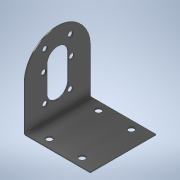
# Autodesk Inventor part: motorBracket
Saved by Autodesk Inventor 2020 (Build 240168000, 168)
## iProperties
Created: 2022-07-22
Part Number: motorBracket
Material: Aluminum 6061
Document SubType Name: Sheet Metal
Designer: iPICLab4
Density: 2.7 g/cm^3
Sheet Metal Rule: Default_mm
Appearance: Dark Gray
Author: iPICLab4
Autodesk Inventor part; units mm, degrees
ref_plane "YZ Plane" through (0, 0, 0) normal (1, 0, 0) x (0, 1, 0)
ref_plane "XZ Plane" through (0, 0, 0) normal (0, 1, 0) x (-1, 0, 0)
ref_plane "XY Plane" through (0, 0, 0) normal (0, 0, 1) x (1, 0, 0)
sketch "Sketch1" plane through (0, 0, 0) normal (0, 1, 0) x (-1, 0, 0)
  line L0 (0, 0) -> (67, 0)
  line L1 (67, -40) -> (0, -40)
  line L2 (0, -40) -> (0, 0)
  line L3 (40, 0) -> (40, -40)
  circle A0 centre (30, -5) radius 1.75
  circle A1 centre (30, -35) radius 1.75
  circle A2 centre (10, -5) radius 1.75
  circle A3 centre (10, -35) radius 1.75
  line L4 (55, -20) -> (70, -20) construction
  line L5 (55, -13.5) -> (70, -13.5)
  line L6 (70, -26.5) -> (55, -26.5)
  arc A4 (55, -13.5) -> (55, -26.5) centre (55, -20) ccw
  arc A5 (70, -26.5) -> (70, -13.5) centre (70, -20) ccw
  circle A6 centre (67, -28.5) radius 1.5
  circle A7 centre (67, -11.5) radius 1.5
  circle A8 centre (50, -27.75) radius 1.5
  circle A9 centre (79, -12.25) radius 1.5
  circle A10 centre (79, -27.75) radius 1.5
  circle A11 centre (50, -12.25) radius 1.5
  arc A12 (67, -40) -> (67, 0) centre (67, -20) ccw
  point P0 (62.5, -20)
  dimension "d1" = 40
  dimension "d2" = 40
  dimension "d3" = 3.5
  dimension "d4" = 3.5
  dimension "d5" = 3.5
  dimension "d6" = 3.5
  dimension "d7" = 30
  dimension "d8" = 30
  dimension "d9" = 5
  dimension "d10" = 5
  dimension "d11" = 10
  dimension "d12" = 10
  dimension "d13" = 10
  dimension "d14" = 10
  dimension "d15" = 3
  dimension "d16" = 3
  dimension "d18" = 3
  dimension "d19" = 17
  dimension "d21" = 3
  dimension "d22" = 3
  dimension "d23" = 3
  dimension "d24" = 15.5
  dimension "d25" = 15.5
  dimension "d26" = 13
  dimension "d27" = 27
  dimension "d28" = 15
  dimension "d30" = 20
  dimension "d31" = 40
  dimension "d32" = 27
  dimension "d33" = 11.5
  dimension "d34" = 27
  dimension "d35" = 12.25
  dimension "d36" = 12.25
  dimension "d37" = 10
  dimension "d38" = 10
  dimension "d39" = 12
  dimension "d40" = 12
  dimension "d43" = 15
  constraints: 16 end point, 13 centre point, 6 point on circle, 5 tangent, 2 horizontal, 2 parallel, 2 point on line, 1 midpoint, 1 vertical
  measures "d1" distance of L1.end L0.start
  measures "d2" distance between parallel lines of L2 L3
  measures "d3" diameter of A0
  measures "d4" diameter of A1
  measures "d5" diameter of A2
  measures "d6" diameter of A3
  measures "d7" distance of A3.centre A2.centre
  measures "d8" distance of A1.centre A0.centre
  measures "d9" distance from line of L1 A1.centre
  measures "d10" distance from line of L1 A3.centre
  measures "d11" distance from line of L2 A3.centre
  measures "d12" distance from line of L2 A2.centre
  measures "d13" distance from line of A0.centre L3
  measures "d14" distance from line of A1.centre L3
  measures "d15" diameter of A6
  measures "d16" diameter of A7
  measures "d18" diameter of A8
  measures "d19" distance of A6.centre A7.centre
  measures "d21" diameter of A9
  measures "d22" diameter of A10
  measures "d23" diameter of A11
  measures "d24" distance between centres of A10 A9
  measures "d25" distance of A8.centre A11.centre
  measures "d26" distance between parallel lines of L6 L5
  measures "d27" distance from line of L3 A7.centre
  measures "d28" distance of L4.start L4.end
  measures "d30" distance between parallel lines of L1 L4
  measures "d31" diameter of A12
  measures "d32" distance from line of L3 A12.centre
  measures "d33" distance from line of L1 A6.centre
  measures "d34" distance from line of L3 A6.centre
  measures "d35" distance from line of L1 A8.centre
  measures "d36" distance from line of L1 A10.centre
  measures "d37" distance from line of L3 A11.centre
  measures "d38" distance from line of L3 A8.centre
  measures "d39" horizontal distance of A7.centre A9.centre
  measures "d40" horizontal distance of A6.centre A10.centre
  measures "d43" distance from line of L4.start L3
extrude "Plate1" add sketch "Sketch1" along normal blind 0.5
fold "Fold1" angle 90 bend radius 0.5 thickness 0.5 k factor 0.44 line from (-40, 0, 0) to (-40, 0, -40) line at bend centre moving side (-1, 0, 0) folds toward (0, 1, 0)
equation "\"d44\" = Thickness"
equation "\"d45\" = BendReliefWidth"
equation "\"d46\" = BendReliefDepth"
equation "\"d47\" = MinimumRemnant"
equation "\"d48\" = TransitionRadius"
equation "\"d50\" = BendRadius"
equation "\"BendRadius\" = Thickness"
equation "\"BendReliefWidth\" = Thickness"
equation "\"BendReliefDepth\" = 0.5 * Thickness"
equation "\"CornerReliefSize\" = 4 * Thickness"
equation "\"MinimumRemnant\" = 2 * Thickness"
equation "\"TransitionRadius\" = BendRadius"
equation "\"JacobiRadiusSize\" = BendRadius"
equation "\"GapSize\" = Thickness"
equation "\"Thickness\" = 0.5"
body "Solid1"
